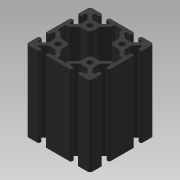
# Autodesk Inventor part: 40-8080
Saved by Autodesk Inventor 2013 (Build 170138000, 138)
## iProperties
Company: 80/20 Inc.
Created: 2014-04-23
Part Number: 40-8080
Material: Generic
Document SubType Name: Modeling
Designer: Ross Bowman
Density: 1 g/cm^3
Engineer: Ross Bowman
Catalog Web Link: 8020.net
Vendor: 80/20 Inc.
Material: 6105-T5 Aluminum
Author: Ross Bowman
Keywords: 80/20 , 8020 , T-Slot , Extrusion
Autodesk Inventor part; units mm, degrees
ref_plane "YZ Plane" through (0, 0, 0) normal (1, 0, 0) x (0, 1, 0)
ref_plane "XZ Plane" through (0, 0, 0) normal (0, 1, 0) x (-1, 0, 0)
ref_plane "XY Plane" through (0, 0, 0) normal (0, 0, 1) x (1, 0, 0)
sketch "Sketch1" plane through (0, 0, 0) normal (0, 0, 1) x (1, 0, 0)
  arc A0 (12.32, 17.07) -> (17.07, 12.32) centre (17.07, 17.07) ccw
  line L0 (22.6578, 12.32) -> (17.07, 12.32)
  arc A1 (26.0165, 10.9288) -> (22.6578, 12.32) centre (22.6578, 7.57) ccw
  line L1 (31.1439, 5.8014) -> (26.0165, 10.9288)
  arc A2 (31.1439, 5.8014) -> (32.0419, 5.4294) centre (32.0419, 6.6994) ccw
  line L2 (34.41, 5.4294) -> (32.0419, 5.4294)
  arc A3 (35.68, 4.1594) -> (34.41, 5.4294) centre (34.41, 4.1594) ccw
  line L3 (35.68, -4.1594) -> (35.68, 4.1594)
  arc A4 (34.41, -5.4294) -> (35.68, -4.1594) centre (34.41, -4.1594) ccw
  line L4 (32.0419, -5.4294) -> (34.41, -5.4294)
  arc A5 (32.0419, -5.4294) -> (31.1439, -5.8014) centre (32.0419, -6.6994) ccw
  line L5 (26.0165, -10.9288) -> (31.1439, -5.8014)
  arc A6 (22.6578, -12.32) -> (26.0165, -10.9288) centre (22.6578, -7.57) ccw
  line L6 (17.07, -12.32) -> (22.6578, -12.32)
  arc A7 (17.07, -12.32) -> (12.32, -17.07) centre (17.07, -17.07) ccw
  line L7 (12.32, -22.6578) -> (12.32, -17.07)
  arc A8 (10.9288, -26.0165) -> (12.32, -22.6578) centre (7.57, -22.6578) ccw
  line L8 (5.8014, -31.1439) -> (10.9288, -26.0165)
  arc A9 (5.8014, -31.1439) -> (5.4294, -32.0419) centre (6.6994, -32.0419) ccw
  line L9 (5.4294, -34.41) -> (5.4294, -32.0419)
  arc A10 (4.1594, -35.68) -> (5.4294, -34.41) centre (4.1594, -34.41) ccw
  line L10 (-4.1594, -35.68) -> (4.1594, -35.68)
  arc A11 (-5.4294, -34.41) -> (-4.1594, -35.68) centre (-4.1594, -34.41) ccw
  line L11 (-5.4294, -32.0419) -> (-5.4294, -34.41)
  arc A12 (-5.4294, -32.0419) -> (-5.8014, -31.1439) centre (-6.6994, -32.0419) ccw
  line L12 (-10.9288, -26.0165) -> (-5.8014, -31.1439)
  arc A13 (-12.32, -22.6578) -> (-10.9288, -26.0165) centre (-7.57, -22.6578) ccw
  line L13 (-12.32, -17.07) -> (-12.32, -22.6578)
  arc A14 (-12.32, -17.07) -> (-17.07, -12.32) centre (-17.07, -17.07) ccw
  line L14 (-22.6578, -12.32) -> (-17.07, -12.32)
  arc A15 (-26.0165, -10.9288) -> (-22.6578, -12.32) centre (-22.6578, -7.57) ccw
  line L15 (-31.1439, -5.8014) -> (-26.0165, -10.9288)
  arc A16 (-31.1439, -5.8014) -> (-32.0419, -5.4294) centre (-32.0419, -6.6994) ccw
  line L16 (-34.41, -5.4294) -> (-32.0419, -5.4294)
  arc A17 (-35.68, -4.1594) -> (-34.41, -5.4294) centre (-34.41, -4.1594) ccw
  line L17 (-35.68, 4.1594) -> (-35.68, -4.1594)
  arc A18 (-34.41, 5.4294) -> (-35.68, 4.1594) centre (-34.41, 4.1594) ccw
  line L18 (-32.0419, 5.4294) -> (-34.41, 5.4294)
  arc A19 (-32.0419, 5.4294) -> (-31.1439, 5.8014) centre (-32.0419, 6.6994) ccw
  line L19 (-26.0165, 10.9288) -> (-31.1439, 5.8014)
  arc A20 (-22.6578, 12.32) -> (-26.0165, 10.9288) centre (-22.6578, 7.57) ccw
  line L20 (-17.07, 12.32) -> (-22.6578, 12.32)
  arc A21 (-17.07, 12.32) -> (-12.32, 17.07) centre (-17.07, 17.07) ccw
  line L21 (-12.32, 22.6578) -> (-12.32, 17.07)
  arc A22 (-10.9288, 26.0165) -> (-12.32, 22.6578) centre (-7.57, 22.6578) ccw
  line L22 (-5.8014, 31.1439) -> (-10.9288, 26.0165)
  arc A23 (-5.8014, 31.1439) -> (-5.4294, 32.0419) centre (-6.6994, 32.0419) ccw
  line L23 (-5.4294, 34.41) -> (-5.4294, 32.0419)
  arc A24 (-4.1594, 35.68) -> (-5.4294, 34.41) centre (-4.1594, 34.41) ccw
  line L24 (4.1594, 35.68) -> (-4.1594, 35.68)
  arc A25 (5.4294, 34.41) -> (4.1594, 35.68) centre (4.1594, 34.41) ccw
  line L25 (5.4294, 32.0419) -> (5.4294, 34.41)
  arc A26 (5.4294, 32.0419) -> (5.8014, 31.1439) centre (6.6994, 32.0419) ccw
  line L26 (10.9288, 26.0165) -> (5.8014, 31.1439)
  arc A27 (12.32, 22.6578) -> (10.9288, 26.0165) centre (7.57, 22.6578) ccw
  line L27 (12.32, 17.07) -> (12.32, 22.6578)
  circle A28 centre (-20, -20) radius 3.4
  circle A29 centre (20, -20) radius 3.4
  circle A30 centre (20, 20) radius 3.4
  circle A31 centre (-20, 20) radius 3.4
  arc A32 (29.0912, 26.0365) -> (27.7, 22.6778) centre (32.45, 22.6778) ccw
  line L28 (29.0912, 26.0365) -> (33.0827, 30.028)
  arc A33 (33.6201, 30.2506) -> (33.0827, 30.028) centre (33.6201, 29.4906) ccw
  line L29 (33.6201, 30.2506) -> (33.9556, 30.2506)
  arc A34 (35.5256, 28.6806) -> (33.9556, 30.2506) centre (33.9556, 28.6806) ccw
  line L30 (35.5256, 28.6806) -> (35.5256, 25.7779)
  arc A35 (35.5256, 25.7779) -> (37.0956, 24.2079) centre (37.0956, 25.7779) ccw
  line L31 (37.0956, 24.2079) -> (38.43, 24.2079)
  arc A36 (38.43, 24.2079) -> (40, 25.7779) centre (38.43, 25.7779) ccw
  line L32 (40, 25.7779) -> (40, 36.83)
  arc A37 (40, 36.83) -> (36.83, 40) centre (36.83, 36.83) ccw
  line L33 (36.83, 40) -> (25.5409, 40)
  arc A38 (25.5409, 40) -> (23.9709, 38.43) centre (25.5409, 38.43) ccw
  line L34 (23.9709, 38.43) -> (23.9709, 37.249)
  arc A39 (23.9709, 37.249) -> (25.5409, 35.679) centre (25.5409, 37.249) ccw
  line L35 (25.5409, 35.679) -> (28.6258, 35.679)
  arc A40 (30.2506, 34.11) -> (28.6258, 35.679) centre (28.6806, 34.11) ccw
  line L36 (30.2506, 34.11) -> (30.2506, 33.6201)
  arc A41 (30.028, 33.0827) -> (30.2506, 33.6201) centre (29.4906, 33.6201) ccw
  line L37 (30.028, 33.0827) -> (26.0365, 29.0912)
  arc A42 (22.6778, 27.7) -> (26.0365, 29.0912) centre (22.6778, 32.45) ccw
  line L38 (22.6778, 27.7) -> (17.3222, 27.7)
  arc A43 (13.9635, 29.0912) -> (17.3222, 27.7) centre (17.3222, 32.45) ccw
  line L39 (13.9635, 29.0912) -> (9.9039, 33.1508)
  arc A44 (9.715, 33.6069) -> (9.9039, 33.1508) centre (10.3601, 33.6069) ccw
  line L40 (9.715, 33.6069) -> (9.715, 34.0968)
  arc A45 (11.2982, 35.68) -> (9.715, 34.0968) centre (11.2982, 34.0968) ccw
  line L41 (11.2982, 35.68) -> (14.6428, 35.68)
  arc A46 (14.6428, 35.68) -> (15.94, 36.9772) centre (14.6428, 36.9772) ccw
  line L42 (15.94, 36.9772) -> (15.94, 38.1948)
  arc A47 (15.94, 38.1948) -> (14.1348, 40) centre (14.1348, 38.1948) ccw
  line L43 (14.1348, 40) -> (-14.1348, 40)
  arc A48 (-14.1348, 40) -> (-15.94, 38.1948) centre (-14.1348, 38.1948) ccw
  line L44 (-15.94, 38.1948) -> (-15.94, 36.9772)
  arc A49 (-15.94, 36.9772) -> (-14.6428, 35.68) centre (-14.6428, 36.9772) ccw
  line L45 (-14.6428, 35.68) -> (-11.2982, 35.68)
  arc A50 (-9.715, 34.0968) -> (-11.2982, 35.68) centre (-11.2982, 34.0968) ccw
  line L46 (-9.715, 34.0968) -> (-9.715, 33.6069)
  arc A51 (-9.9039, 33.1508) -> (-9.715, 33.6069) centre (-10.3601, 33.6069) ccw
  line L47 (-9.9039, 33.1508) -> (-13.9635, 29.0912)
  arc A52 (-17.3222, 27.7) -> (-13.9635, 29.0912) centre (-17.3222, 32.45) ccw
  line L48 (-17.3222, 27.7) -> (-22.6778, 27.7)
  arc A53 (-26.0365, 29.0912) -> (-22.6778, 27.7) centre (-22.6778, 32.45) ccw
  line L49 (-26.0365, 29.0912) -> (-30.0961, 33.1508)
  arc A54 (-30.285, 33.6069) -> (-30.0961, 33.1508) centre (-29.6399, 33.6069) ccw
  line L50 (-30.285, 33.6069) -> (-30.285, 34.0968)
  arc A55 (-28.7018, 35.68) -> (-30.285, 34.0968) centre (-28.7018, 34.0968) ccw
  line L51 (-28.7018, 35.68) -> (-25.3572, 35.68)
  arc A56 (-25.3572, 35.68) -> (-24.06, 36.9772) centre (-25.3572, 36.9772) ccw
  line L52 (-24.06, 36.9772) -> (-24.06, 38.1948)
  arc A57 (-24.06, 38.1948) -> (-25.8652, 40) centre (-25.8652, 38.1948) ccw
  line L53 (-25.8652, 40) -> (-36.83, 40)
  arc A58 (-36.83, 40) -> (-40, 36.83) centre (-36.83, 36.83) ccw
  line L54 (-40, 36.83) -> (-40, 25.8652)
  arc A59 (-40, 25.8652) -> (-38.1948, 24.06) centre (-38.1948, 25.8652) ccw
  line L55 (-38.1948, 24.06) -> (-36.9772, 24.06)
  arc A60 (-36.9772, 24.06) -> (-35.68, 25.3572) centre (-36.9772, 25.3572) ccw
  line L56 (-35.68, 25.3572) -> (-35.68, 28.6806)
  arc A61 (-34.11, 30.2506) -> (-35.68, 28.6806) centre (-34.11, 28.6806) ccw
  line L57 (-34.11, 30.2506) -> (-33.6201, 30.2506)
  arc A62 (-33.0827, 30.028) -> (-33.6201, 30.2506) centre (-33.6201, 29.4906) ccw
  line L58 (-33.0827, 30.028) -> (-29.0912, 26.0365)
  arc A63 (-27.7, 22.6778) -> (-29.0912, 26.0365) centre (-32.45, 22.6778) ccw
  line L59 (-27.7, 22.6778) -> (-27.7, 17.3222)
  arc A64 (-29.0912, 13.9635) -> (-27.7, 17.3222) centre (-32.45, 17.3222) ccw
  line L60 (-29.0912, 13.9635) -> (-33.0827, 9.972)
  arc A65 (-33.6201, 9.7494) -> (-33.0827, 9.972) centre (-33.6201, 10.5094) ccw
  line L61 (-33.6201, 9.7494) -> (-34.11, 9.7494)
  arc A66 (-35.68, 11.3194) -> (-34.11, 9.7494) centre (-34.11, 11.3194) ccw
  line L62 (-35.68, 11.3194) -> (-35.68, 14.6428)
  arc A67 (-35.68, 14.6428) -> (-36.9772, 15.94) centre (-36.9772, 14.6428) ccw
  line L63 (-36.9772, 15.94) -> (-38.1948, 15.94)
  arc A68 (-38.1948, 15.94) -> (-40, 14.1348) centre (-38.1948, 14.1348) ccw
  line L64 (-40, 14.1348) -> (-40, -14.4473)
  arc A69 (-40, -14.4473) -> (-38.43, -16.0173) centre (-38.43, -14.4473) ccw
  line L65 (-38.43, -16.0173) -> (-37.25, -16.0173)
  arc A70 (-37.25, -16.0173) -> (-35.68, -14.4473) centre (-37.25, -14.4473) ccw
  line L66 (-35.68, -14.4473) -> (-35.68, -11.3194)
  arc A71 (-34.11, -9.7494) -> (-35.68, -11.3194) centre (-34.11, -11.3194) ccw
  line L67 (-34.11, -9.7494) -> (-33.6201, -9.7494)
  arc A72 (-33.0827, -9.972) -> (-33.6201, -9.7494) centre (-33.6201, -10.5094) ccw
  line L68 (-33.0827, -9.972) -> (-29.0912, -13.9635)
  arc A73 (-27.7, -17.3222) -> (-29.0912, -13.9635) centre (-32.45, -17.3222) ccw
  line L69 (-27.7, -17.3222) -> (-27.7, -22.6778)
  arc A74 (-29.0912, -26.0365) -> (-27.7, -22.6778) centre (-32.45, -22.6778) ccw
  line L70 (-29.0912, -26.0365) -> (-32.8718, -29.8171)
  arc A75 (-33.3827, -30.0392) -> (-32.8718, -29.8171) centre (-33.4092, -29.2797) ccw
  line L71 (-33.3827, -30.0392) -> (-34.0552, -30.0627)
  arc A76 (-35.68, -28.4937) -> (-34.0552, -30.0627) centre (-34.11, -28.4937) ccw
  line L72 (-35.68, -28.4937) -> (-35.68, -25.591)
  arc A77 (-35.68, -25.591) -> (-37.25, -24.021) centre (-37.25, -25.591) ccw
  line L73 (-37.25, -24.021) -> (-38.43, -24.021)
  arc A78 (-38.43, -24.021) -> (-40, -25.591) centre (-38.43, -25.591) ccw
  line L74 (-40, -25.591) -> (-40, -36.83)
  arc A79 (-40, -36.83) -> (-36.83, -40) centre (-36.83, -36.83) ccw
  line L75 (-36.83, -40) -> (-25.7231, -40)
  arc A80 (-25.7231, -40) -> (-24.1531, -38.43) centre (-25.7231, -38.43) ccw
  line L76 (-24.1531, -38.43) -> (-24.1531, -37.25)
  arc A81 (-24.1531, -37.25) -> (-25.7231, -35.68) centre (-25.7231, -37.25) ccw
  line L77 (-25.7231, -35.68) -> (-28.6806, -35.68)
  arc A82 (-30.2506, -34.11) -> (-28.6806, -35.68) centre (-28.6806, -34.11) ccw
  line L78 (-30.2506, -34.11) -> (-30.2506, -33.6201)
  arc A83 (-30.028, -33.0827) -> (-30.2506, -33.6201) centre (-29.4906, -33.6201) ccw
  line L79 (-30.028, -33.0827) -> (-26.0365, -29.0912)
  arc A84 (-22.6778, -27.7) -> (-26.0365, -29.0912) centre (-22.6778, -32.45) ccw
  line L80 (-22.6778, -27.7) -> (-17.3222, -27.7)
  arc A85 (-13.9635, -29.0912) -> (-17.3222, -27.7) centre (-17.3222, -32.45) ccw
  line L81 (-13.9635, -29.0912) -> (-10.2038, -32.8509)
  arc A86 (-9.9816, -33.3618) -> (-10.2038, -32.8509) centre (-10.7412, -33.3883) ccw
  line L82 (-9.9816, -33.3618) -> (-9.9574, -34.0552)
  arc A87 (-11.5265, -35.68) -> (-9.9574, -34.0552) centre (-11.5265, -34.11) ccw
  line L83 (-11.5265, -35.68) -> (-14.4292, -35.68)
  arc A88 (-14.4292, -35.68) -> (-15.9992, -37.25) centre (-14.4292, -37.25) ccw
  line L84 (-15.9992, -37.25) -> (-15.9992, -38.43)
  arc A89 (-15.9992, -38.43) -> (-14.4292, -40) centre (-14.4292, -38.43) ccw
  line L85 (-14.4292, -40) -> (14.4246, -40)
  arc A90 (14.4246, -40) -> (15.9946, -38.43) centre (14.4246, -38.43) ccw
  line L86 (15.9946, -38.43) -> (15.9946, -37.0326)
  arc A91 (15.9946, -37.0326) -> (14.4246, -35.4626) centre (14.4246, -37.0326) ccw
  line L87 (14.4246, -35.4626) -> (11.3824, -35.4626)
  arc A92 (9.8124, -33.8926) -> (11.3824, -35.4626) centre (11.3824, -33.8926) ccw
  line L88 (9.8124, -33.8926) -> (9.8124, -33.5571)
  arc A93 (10.035, -33.0197) -> (9.8124, -33.5571) centre (10.5724, -33.5571) ccw
  line L89 (10.035, -33.0197) -> (13.9635, -29.0912)
  arc A94 (17.3222, -27.7) -> (13.9635, -29.0912) centre (17.3222, -32.45) ccw
  line L90 (17.3222, -27.7) -> (22.6778, -27.7)
  arc A95 (26.0365, -29.0912) -> (22.6778, -27.7) centre (22.6778, -32.45) ccw
  line L91 (26.0365, -29.0912) -> (29.7949, -32.8496)
  arc A96 (30.0171, -33.3605) -> (29.7949, -32.8496) centre (29.2575, -33.387) ccw
  line L92 (30.0171, -33.3605) -> (30.0413, -34.0552)
  arc A97 (28.4723, -35.68) -> (30.0413, -34.0552) centre (28.4723, -34.11) ccw
  line L93 (28.4723, -35.68) -> (25.5696, -35.68)
  arc A98 (25.5696, -35.68) -> (23.9996, -37.25) centre (25.5696, -37.25) ccw
  line L94 (23.9996, -37.25) -> (23.9996, -38.43)
  arc A99 (23.9996, -38.43) -> (25.5696, -40) centre (25.5696, -38.43) ccw
  line L95 (25.5696, -40) -> (36.83, -40)
  arc A100 (36.83, -40) -> (40, -36.83) centre (36.83, -36.83) ccw
  line L96 (40, -36.83) -> (40, -25.7779)
  arc A101 (40, -25.7779) -> (38.43, -24.2079) centre (38.43, -25.7779) ccw
  line L97 (38.43, -24.2079) -> (37.25, -24.2079)
  arc A102 (37.25, -24.2079) -> (35.68, -25.7779) centre (37.25, -25.7779) ccw
  line L98 (35.68, -25.7779) -> (35.68, -28.6806)
  arc A103 (34.11, -30.2506) -> (35.68, -28.6806) centre (34.11, -28.6806) ccw
  line L99 (34.11, -30.2506) -> (33.6201, -30.2506)
  arc A104 (33.0827, -30.028) -> (33.6201, -30.2506) centre (33.6201, -29.4906) ccw
  line L100 (33.0827, -30.028) -> (29.0912, -26.0365)
  arc A105 (27.7, -22.6778) -> (29.0912, -26.0365) centre (32.45, -22.6778) ccw
  line L101 (27.7, -22.6778) -> (27.7, -17.3222)
  arc A106 (29.0912, -13.9635) -> (27.7, -17.3222) centre (32.45, -17.3222) ccw
  line L102 (29.0912, -13.9635) -> (33.0827, -9.972)
  arc A107 (33.6201, -9.7494) -> (33.0827, -9.972) centre (33.6201, -10.5094) ccw
  line L103 (33.6201, -9.7494) -> (34.11, -9.7494)
  arc A108 (35.68, -11.3194) -> (34.11, -9.7494) centre (34.11, -11.3194) ccw
  line L104 (35.68, -11.3194) -> (35.68, -14.2221)
  arc A109 (35.68, -14.2221) -> (37.25, -15.7921) centre (37.25, -14.2221) ccw
  line L105 (37.25, -15.7921) -> (38.43, -15.7921)
  arc A110 (38.43, -15.7921) -> (40, -14.2221) centre (38.43, -14.2221) ccw
  line L106 (40, -14.2221) -> (40, 14.2221)
  arc A111 (40, 14.2221) -> (38.43, 15.7921) centre (38.43, 14.2221) ccw
  line L107 (38.43, 15.7921) -> (37.25, 15.7921)
  arc A112 (37.25, 15.7921) -> (35.68, 14.2221) centre (37.25, 14.2221) ccw
  line L108 (35.68, 14.2221) -> (35.68, 11.3194)
  arc A113 (34.11, 9.7494) -> (35.68, 11.3194) centre (34.11, 11.3194) ccw
  line L109 (34.11, 9.7494) -> (33.6201, 9.7494)
  arc A114 (33.0827, 9.972) -> (33.6201, 9.7494) centre (33.6201, 10.5094) ccw
  line L110 (33.0827, 9.972) -> (29.0912, 13.9635)
  arc A115 (27.7, 17.3222) -> (29.0912, 13.9635) centre (32.45, 17.3222) ccw
  line L111 (27.7, 17.3222) -> (27.7, 22.6778)
  point P0 (0, 0)
  constraints: 224 end point, 224 point on circle, 116 centre point
extrude "Extrusion1" add sketch "Sketch1" against normal blind 100
body "Solid1"
